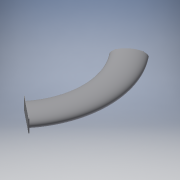
# Autodesk Inventor part: Handle bars holder
Saved by Autodesk Inventor 2018 (Build 220112000, 112)
## iProperties
Created: 2018-08-14
Part Number: Handle bars holder
Material: Generic
Document SubType Name: Modeling
Designer: ruben
Density: 1 g/cm^3
Sheet Metal Rule: Default_mm
Appearance: Default
Author: ruben
Autodesk Inventor part; units mm, degrees
ref_plane "YZ Plane" through (0, 0, 0) normal (1, 0, 0) x (0, 1, 0)
sketch "Sketch3" plane through (0, 0, 0) normal (0, 0, 1) x (1, 0, 0)
  line L0 (-140, 0) -> (140, 0) projected
  line L1 (0, -157.4286) -> (0, 67.0714) projected
  arc A0 (100, 0) -> (-100, 0) centre (0, -125.3571) ccw
  line L2 (-90.9685, 35) -> (88.04, 35) construction
  point P0 (0, 0)
  point P1 (0, 35)
  dimension "d0" = 200
  dimension "d1" = 35
  constraints: 3 point on circle, 3 point on line, 2 end point, 1 centre point, 1 parallel, 1 symmetric about line
  measures "d0" distance of A0.start A0.end
  measures "d1" distance from line of L0 point (0, 35)
ref_plane "Work Plane1" through (100, 0, 0) normal (-0.7817, 0.6236, 0) x (-0.6236, -0.7817, 0)
sketch "Sketch5" plane through (100, 0, 0) normal (-0.7817, 0.6236, 0) x (-0.6236, -0.7817, 0)
  ellipse E0 centre (0, 0) end of major axis (0, -12.5) minor radius 27.5
  ellipse E1 centre (0, 0) end of major axis (0, -10.5) minor radius 25.5
  point P0 (62.3608, 0)
  dimension "d2" = 27.5
  dimension "d3" = 12.5
  dimension "d4" = 25.5
  dimension "d5" = 10.5
  constraints: 1 coincident, 4 other
sweep "Sweep1" add profiles "Sketch5" path "Sketch3" path curves A0
sketch "Sketch6" plane through (100, 0, 0) normal (-0.7817, 0.6236, 0) x (-0.6236, -0.7817, 0)
  line L0 (27.5, 12.5) -> (-27.5, 12.5)
  line L1 (-27.5, 12.5) -> (-27.5, -12.5)
  line L2 (-27.5, -12.5) -> (27.5, -12.5)
  line L3 (27.5, -12.5) -> (27.5, 12.5)
  line L4 (27.5, 12.5) -> (-27.5, -12.5) construction
  line L5 (-27.5, 12.5) -> (27.5, -12.5) construction
  point P0 (62.3608, 0)
  point P1 (0, 0)
  dimension "d8" = 55
  dimension "d9" = 25
  constraints: 12 end point, 2 midpoint, 2 parallel, 1 horizontal, 1 perpendicular
  measures "d8" distance of L2.end L1.end
  measures "d9" distance of L1.end L0.end
extrude "Extrusion1" add sketch "Sketch6" against normal blind 1
ref_plane "Work Plane2" through (-100, 0, 0) normal (-0.7817, -0.6236, 0) x (0, 0, 1)
sketch "Sketch7" plane through (-100, 0, 0) normal (-0.7817, -0.6236, 0) x (0, 0, 1)
  line L0 (-7.5, -20) -> (7.5, -20)
  line L1 (7.5, -20) -> (7.5, 20)
  line L2 (7.5, 20) -> (-7.5, 20)
  line L3 (-7.5, 20) -> (-7.5, -20)
  line L4 (-7.5, -20) -> (7.5, 20) construction
  line L5 (7.5, -20) -> (-7.5, 20) construction
  point P0 (0, -62.3608)
  point P1 (0, 0)
  dimension "d12" = 15
  dimension "d13" = 40
  constraints: 12 end point, 2 midpoint, 2 parallel, 1 horizontal, 1 perpendicular
  measures "d12" distance of L2.end L1.end
  measures "d13" distance of L1.end L0.end
extrude "Extrusion2" add sketch "Sketch7" along normal blind 3
equation "\"BendRadius\" = Thickness"
equation "\"BendReliefWidth\" = Thickness"
equation "\"BendReliefDepth\" = 0.5 * Thickness"
equation "\"CornerReliefSize\" = 4 * Thickness"
equation "\"MinimumRemnant\" = 2 * Thickness"
equation "\"TransitionRadius\" = BendRadius"
equation "\"JacobiRadiusSize\" = BendRadius"
equation "\"GapSize\" = Thickness"
equation "\"Thickness\" = 0.5"
body "Solid1"
